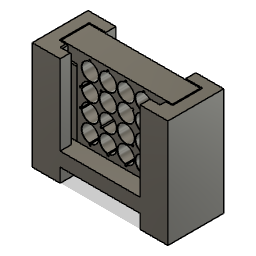
Prototype30 (Autodesk Fusion 360 design; units mm, degrees)
Autodesk Fusion 360 part; units mm, degrees
sketch "Esquisse1" plane through (0, 0, 0) normal (0, 0, 1) x (1, 0, 0) in component "Support_electroaimant"
  circle A0 centre (-16.1, 48.3478) radius 15.1
  line L0 (-14.9, 66.6) -> (-17.3, 66.6) construction
  line L1 (-17.3, 66.6) -> (-17.3, 63.4) construction
  line L2 (-17.3, 63.4) -> (-14.9, 63.4) construction
  line L3 (-14.9, 63.4) -> (-14.9, 66.6) construction
  line L4 (-14.9, 63.4) -> (-14.9, 66.6)
  line L5 (-17.3, 66.6) -> (-17.3, 63.4)
  line L6 (-14.9, 66.6) -> (-17.3, 66.6)
  line L7 (0, 71.8) -> (0, -71.8) construction
  line L8 (71.8, 71.8) -> (-71.8, 71.8)
  line L9 (-71.8, 71.8) -> (-71.8, -71.8)
  line L10 (-71.8, -71.8) -> (71.8, -71.8)
  line L11 (71.8, -71.8) -> (71.8, 71.8)
  line L12 (71.8, 71.8) -> (-71.8, -71.8) construction
  line L13 (-71.8, 71.8) -> (71.8, -71.8) construction
  line L14 (17.3, 63.4) -> (14.9, 63.4) construction
  line L15 (17.3, 66.6) -> (17.3, 63.4)
  line L16 (14.9, 66.6) -> (17.3, 66.6) construction
  line L17 (17.3, 66.6) -> (17.3, 63.4) construction
  line L18 (14.9, 63.4) -> (14.9, 66.6) construction
  line L19 (14.9, 63.4) -> (14.9, 66.6)
  line L20 (14.9, 66.6) -> (17.3, 66.6)
  circle A1 centre (16.1, 48.3478) radius 15.1
  line L21 (-32.2, 71.8) -> (-32.2, -71.8) construction
  line L22 (-47.1, 63.4) -> (-49.5, 63.4) construction
  line L23 (-49.5, 66.6) -> (-47.1, 66.6)
  line L24 (-47.1, 66.6) -> (-47.1, 63.4) construction
  circle A2 centre (-48.3, 48.3478) radius 15.1
  line L25 (-47.1, 66.6) -> (-47.1, 63.4)
  line L26 (-49.5, 63.4) -> (-49.5, 66.6)
  line L27 (-49.5, 63.4) -> (-49.5, 66.6) construction
  line L28 (-49.5, 66.6) -> (-47.1, 66.6) construction
  line L29 (32.2, 71.8) -> (32.2, -71.8) construction
  circle A3 centre (48.3, 48.3478) radius 15.1
  line L30 (49.5, 63.4) -> (49.5, 66.6) construction
  line L31 (47.1, 66.6) -> (47.1, 63.4)
  line L32 (49.5, 66.6) -> (47.1, 66.6) construction
  line L33 (47.1, 66.6) -> (47.1, 63.4) construction
  line L34 (47.1, 63.4) -> (49.5, 63.4) construction
  line L35 (49.5, 63.4) -> (49.5, 66.6)
  line L36 (49.5, 66.6) -> (47.1, 66.6)
  line L37 (-71.8, 0) -> (71.8, 0) construction
  circle A4 centre (-16.1, -48.3478) radius 15.1
  line L38 (-14.9, -66.6) -> (-17.3, -66.6)
  line L39 (-14.9, -63.4) -> (-14.9, -66.6)
  line L40 (47.1, -66.6) -> (47.1, -63.4)
  line L41 (47.1, -63.4) -> (49.5, -63.4) construction
  line L42 (-49.5, -66.6) -> (-47.1, -66.6)
  line L43 (17.3, -66.6) -> (17.3, -63.4) construction
  line L44 (17.3, -66.6) -> (17.3, -63.4)
  line L45 (14.9, -63.4) -> (14.9, -66.6) construction
  circle A5 centre (48.3, -48.3478) radius 15.1
  line L46 (49.5, -66.6) -> (47.1, -66.6)
  line L47 (49.5, -66.6) -> (47.1, -66.6) construction
  line L48 (17.3, -63.4) -> (14.9, -63.4) construction
  line L49 (-49.5, -63.4) -> (-49.5, -66.6) construction
  circle A6 centre (-48.3, -48.3478) radius 15.1
  circle A7 centre (16.1, -48.3478) radius 15.1
  line L50 (14.9, -63.4) -> (14.9, -66.6)
  line L51 (14.9, -66.6) -> (17.3, -66.6) construction
  line L52 (-49.5, -63.4) -> (-49.5, -66.6)
  line L53 (49.5, -63.4) -> (49.5, -66.6)
  line L54 (49.5, -63.4) -> (49.5, -66.6) construction
  line L55 (-17.3, -63.4) -> (-14.9, -63.4) construction
  line L56 (-14.9, -66.6) -> (-17.3, -66.6) construction
  line L57 (-49.5, -66.6) -> (-47.1, -66.6) construction
  line L58 (-47.1, -66.6) -> (-47.1, -63.4)
  line L59 (47.1, -66.6) -> (47.1, -63.4) construction
  line L60 (-14.9, -63.4) -> (-14.9, -66.6) construction
  line L61 (-17.3, -66.6) -> (-17.3, -63.4)
  line L62 (-47.1, -66.6) -> (-47.1, -63.4) construction
  line L63 (-17.3, -66.6) -> (-17.3, -63.4) construction
  line L64 (14.9, -66.6) -> (17.3, -66.6)
  line L65 (-47.1, -63.4) -> (-49.5, -63.4) construction
  line L66 (-71.8, 32.2478) -> (71.8, 32.2478) construction
  line L67 (-66.5522, 14.9478) -> (-63.3522, 14.9478) construction
  line L68 (-63.3522, 17.3478) -> (-66.5522, 17.3478) construction
  line L69 (-66.5522, 17.3478) -> (-66.5522, 14.9478) construction
  line L70 (-27.5921, 25.9428) -> (-29.8548, 28.2055)
  line L71 (-66.5522, 14.9478) -> (-63.3522, 14.9478)
  circle A8 centre (-16.1, 16.1478) radius 15.1
  line L72 (-63.3522, 17.3478) -> (-66.5522, 17.3478)
  line L73 (-25.895, 27.6398) -> (-27.5921, 25.9428) construction
  line L74 (-66.5522, 17.3478) -> (-66.5522, 14.9478)
  line L75 (-28.1578, 29.9026) -> (-25.895, 27.6398) construction
  line L76 (-29.8548, 28.2055) -> (-28.1578, 29.9026) construction
  line L77 (-63.3522, 14.9478) -> (-63.3522, 17.3478) construction
  line L78 (-27.5921, 25.9428) -> (-29.8548, 28.2055) construction
  circle A9 centre (-48.3, 16.1478) radius 15.1
  line L79 (-28.1578, 29.9026) -> (-25.895, 27.6398)
  line L80 (-29.8548, 28.2055) -> (-28.1578, 29.9026)
  line L81 (29.8548, 28.2055) -> (28.1578, 29.9026) construction
  line L82 (66.5522, 14.9478) -> (63.3522, 14.9478) construction
  line L83 (66.5522, 14.9478) -> (63.3522, 14.9478)
  circle A10 centre (48.3, 16.1478) radius 15.1
  line L84 (66.5522, 17.3478) -> (66.5522, 14.9478)
  line L85 (63.3522, 17.3478) -> (66.5522, 17.3478)
  line L86 (25.895, 27.6398) -> (27.5921, 25.9428) construction
  line L87 (27.5921, 25.9428) -> (29.8548, 28.2055) construction
  line L88 (28.1578, 29.9026) -> (25.895, 27.6398)
  line L89 (63.3522, 17.3478) -> (66.5522, 17.3478) construction
  circle A11 centre (16.1, 16.1478) radius 15.1
  line L90 (63.3522, 14.9478) -> (63.3522, 17.3478) construction
  line L91 (29.8548, 28.2055) -> (28.1578, 29.9026)
  line L92 (27.5921, 25.9428) -> (29.8548, 28.2055)
  line L93 (66.5522, 17.3478) -> (66.5522, 14.9478) construction
  line L94 (28.1578, 29.9026) -> (25.895, 27.6398) construction
  line L95 (66.5522, -17.3478) -> (66.5522, -14.9478) construction
  line L96 (-66.5522, -17.3478) -> (-66.5522, -14.9478) construction
  line L97 (-29.8548, -28.2055) -> (-28.1578, -29.9026)
  line L98 (-29.8548, -28.2055) -> (-28.1578, -29.9026) construction
  line L99 (-63.3522, -17.3478) -> (-66.5522, -17.3478)
  line L100 (-63.3522, -14.9478) -> (-63.3522, -17.3478) construction
  line L101 (-63.3522, -17.3478) -> (-66.5522, -17.3478) construction
  line L102 (-28.1578, -29.9026) -> (-25.895, -27.6398) construction
  line L103 (-66.5522, -17.3478) -> (-66.5522, -14.9478)
  line L104 (-25.895, -27.6398) -> (-27.5921, -25.9428) construction
  line L105 (29.8548, -28.2055) -> (28.1578, -29.9026)
  circle A12 centre (-48.3, -16.1478) radius 15.1
  line L106 (29.8548, -28.2055) -> (28.1578, -29.9026) construction
  line L107 (-66.5522, -14.9478) -> (-63.3522, -14.9478) construction
  line L108 (-27.5921, -25.9428) -> (-29.8548, -28.2055) construction
  circle A13 centre (-16.1, -16.1478) radius 15.1
  line L109 (-28.1578, -29.9026) -> (-25.895, -27.6398)
  line L110 (-27.5921, -25.9428) -> (-29.8548, -28.2055)
  line L111 (-66.5522, -14.9478) -> (-63.3522, -14.9478)
  line L112 (66.5522, -14.9478) -> (63.3522, -14.9478)
  line L113 (63.3522, -17.3478) -> (66.5522, -17.3478)
  line L114 (66.5522, -14.9478) -> (63.3522, -14.9478) construction
  line L115 (27.5921, -25.9428) -> (29.8548, -28.2055)
  circle A14 centre (16.1, -16.1478) radius 15.1
  line L116 (28.1578, -29.9026) -> (25.895, -27.6398)
  line L117 (63.3522, -17.3478) -> (66.5522, -17.3478) construction
  line L118 (25.895, -27.6398) -> (27.5921, -25.9428) construction
  circle A15 centre (48.3, -16.1478) radius 15.1
  line L119 (63.3522, -14.9478) -> (63.3522, -17.3478) construction
  line L120 (66.5522, -17.3478) -> (66.5522, -14.9478)
  line L121 (28.1578, -29.9026) -> (25.895, -27.6398) construction
  line L122 (27.5921, -25.9428) -> (29.8548, -28.2055) construction
  point P0 (-17.3, 63.4)
  point P1 (-14.9, 63.4)
  point P2 (-16.1, 66.6)
  point P3 (14.9, 63.4)
  point P4 (17.3, 63.4)
  point P5 (-1, 48.3478)
  point P6 (1, 48.3478)
  point P7 (-49.5, 63.4)
  point P8 (-47.1, 63.4)
  point P9 (-48.3, 66.6)
  point P10 (47.1, 63.4)
  point P11 (49.5, 63.4)
  point P12 (-63.4, -48.3478)
  point P13 (17.3, -63.4)
  point P14 (-48.3, -66.6)
  point P15 (49.5, -63.4)
  point P16 (14.9, -63.4)
  point P17 (-31.2, -48.3478)
  point P18 (1, -48.3478)
  point P19 (-16.1, -66.6)
  point P20 (-47.1, -63.4)
  point P21 (-1, -48.3478)
  point P22 (-14.9, -63.4)
  point P23 (-49.5, -63.4)
  point P24 (33.2, -48.3478)
  point P25 (31.2, -48.3478)
  point P26 (47.1, -63.4)
  point P27 (-17.3, -63.4)
  point P28 (-66.5522, 16.1478)
  point P29 (-63.3522, 14.9478)
  point P30 (-27.5921, 25.9428)
  point P31 (-29.0063, 29.054)
  point P32 (-25.895, 27.6398)
  point P33 (-63.3522, 17.3478)
  point P34 (27.5921, 25.9428)
  point P35 (66.5522, 16.1478)
  point P36 (63.3522, 14.9478)
  point P37 (63.3522, 17.3478)
  point P38 (71.8, 32.2478)
  point P39 (25.895, 27.6398)
  point P40 (29.0063, 29.054)
  point P41 (-25.895, -27.6398)
  point P42 (63.3522, -14.9478)
  point P43 (27.5921, -25.9428)
  point P44 (-66.5522, -16.1478)
  point P45 (25.895, -27.6398)
  point P46 (-63.3522, -14.9478)
  point P47 (-27.5921, -25.9428)
  point P48 (-63.3522, -17.3478)
  point P49 (63.3522, -17.3478)
  point P50 (66.5522, -16.1478)
  point P51 (-29.0063, -29.054)
  point P52 (29.0063, -29.054)
  dimension "d1" = 30.2
  dimension "d4" = 2.4
  dimension "d5" = 3.2
  dimension "d8" = 143.6
  dimension "d9" = 143.6
  dimension "d11" = 2
  dimension "d17" = 32.2
  dimension "d18" = 32.2
  dimension "d19" = 16.1
  constraint horizontal L0
  constraint vertical L1
  constraint horizontal L2
  constraint vertical L3
  constraint coincident P0 L1.end
  constraint coincident P1 L2.end
  constraint coincident A0 P0
  constraint coincident A0 P1
  constraint vertical L7
  constraint coincident origin L7
  constraint perpendicular L8 L9
  constraint parallel L8 L10
  constraint parallel L9 L11
  constraint coincident L12 origin
  constraint coincident L13 origin
  constraint midpoint L0 P2
  constraint symmetric A0 L7 A1
  constraint symmetric L0.start L7 L16.start
  constraint symmetric L0.end L7 L15.start
  constraint symmetric P0 L7 L14.start
  constraint symmetric P1 L7 P3
  constraint symmetric P0 L7 P4
  constraint coincident A0 P5
  constraint coincident A1 P6
  constraint vertical L21
  constraint symmetric A0 L21 A2
  constraint symmetric L0.start L21 L23.start
  constraint symmetric L0.end L21 L23.end
  constraint symmetric P0 L21 P8
  constraint symmetric P1 L21 P7
  constraint symmetric P1 L21 L22.end
  constraint symmetric P2 L21 P9
  constraint coincident L8 L21.start
  constraint coincident L10 L21.end
  constraint coincident L8 L29.start
  constraint coincident L10 L29.end
  constraint symmetric P3 L29 P11
  constraint symmetric P4 L29 P10
  constraint symmetric L15.start L29 L31.start
  constraint symmetric L16.start L29 L30.end
  constraint symmetric A1 L29 A3
  constraint symmetric A0 L37 A4
  constraint symmetric L0.start L37 L38.start
  constraint symmetric L0.end L37 L38.end
  constraint symmetric P0 L37 P27
  constraint symmetric P1 L37 P22
  constraint symmetric P2 L37 P19
  constraint symmetric P3 L37 L45.start
  constraint symmetric P4 L37 P13
  constraint symmetric P3 L37 P16
  constraint symmetric L15.start L37 L43.start
  constraint symmetric L16.start L37 L45.end
  constraint symmetric A1 L37 A7
  constraint symmetric P5 L37 P21
  constraint symmetric P6 L37 P18
  constraint symmetric P7 L37 P23
  constraint symmetric L23.end L37 L42.end
  constraint symmetric P8 L37 P20
  constraint symmetric P9 L37 P14
  constraint symmetric L23.start L37 L42.start
  constraint symmetric A2 L37 A6
  constraint symmetric P10 L37 P26
  constraint symmetric L30.end L37 L46.start
  constraint symmetric P11 L37 P15
  constraint symmetric L31.start L37 L40.start
  constraint symmetric A3 L37 A5
  constraint coincident L9 L66.start
  constraint coincident L11 P38
  constraint symmetric L7 L66.start P38
  constraint symmetric L7 L70.end L81.start
  constraint symmetric L7 L68.end L84.start
  constraint symmetric L7 P28 P35
  constraint symmetric L7 P29 P36
  constraint symmetric L7 P32 P39
  constraint symmetric L7 P33 P37
  constraint symmetric L7 L75.start L81.end
  constraint symmetric L7 P30 P34
  constraint symmetric L7 L67.start L82.start
  constraint symmetric L7 P31 P40
  constraint symmetric L7 A8 A11
  constraint symmetric L7 A9 A10
  constraint symmetric L37 L70.end L97.start
  constraint symmetric L37 L68.end L96.start
  constraint symmetric L37 P28 P44
  constraint symmetric L37 P29 P46
  constraint symmetric L37 P32 P41
  constraint symmetric L37 P33 P48
  constraint symmetric L37 L75.start L97.end
  constraint symmetric L37 P30 P47
  constraint symmetric L37 L67.start L96.end
  constraint symmetric L37 P31 P51
  constraint symmetric L37 A8 A13
  constraint symmetric L37 A9 A12
  constraint symmetric L37 P34 P43
  constraint symmetric L37 P36 P42
  constraint symmetric L37 P35 P50
  constraint symmetric L37 L82.start L95.end
  constraint symmetric L37 P37 P49
  constraint symmetric L37 L84.start L95.start
  constraint symmetric L37 L81.start L105.start
  constraint symmetric L37 P39 P45
  constraint symmetric L37 L81.end L105.end
  constraint symmetric L37 P40 P52
  constraint symmetric L37 A10 A15
  constraint symmetric L37 A11 A14
  measures "d1" diameter of A0
  measures "d4" distance of L0.start L0.end
  measures "d5" distance of L0.start P1
  measures "d8" distance of L8.end L9.end
  measures "d9" distance of L8.start L8.end
  measures "d11" distance of P5 P6
  measures "d17" distance of A0.centre A2.centre
  measures "d18" distance of A1.centre A3.centre
  measures "d19" distance of A2.centre L66
extrude "Extrusion2" add sketch "Esquisse1" against normal blind 25 contours A0 | L8 L9 L10 L11 | A1 | A2 | A3 | A4 | A5 | A6 | A7 | A8 | A9 | A10 | A11 | A13 | A12 | A14 | A15 makes body 1 in component "Support_electroaimant"
extrude "Extrusion1" add sketch "Esquisse1" along normal blind 25 bodies 1 in component "Support_electroaimant"
chamfer "Chanfrein1" distance 0.4 angle 45 64 edges at (-48.3, 66.6, 25) (-49.5, 65, 25) (-47.1, 65, 25) (-48.3, 33.2478, 25) (-16.1, 33.2478, 25) (-14.9, 65, 25) (-16.1, 66.6, 25) (-17.3, 65, 25) (16.1, 33.2478, 25) (14.9, 65, 25) (16.1, 66.6, 25) (17.3, 65, 25) (48.3, 33.2478, 25) (47.1, 65, 25) (48.3, 66.6, 25) (49.5, 65, 25) (33.2, 16.1478, 25) (64.9522, 17.3478, 25) (66.5522, 16.1478, 25) (64.9522, 14.9478, 25) (29.0063, 29.054, 25) (28.7234, 27.0741, 25) (27.0264, 28.7712, 25) (5.4227, 5.4704, 25) (-5.4227, 5.4704, 25) (-27.0264, 28.7712, 25) (-29.0063, 29.054, 25) (-28.7234, 27.0741, 25) (-33.2, 16.1478, 25) (-64.9522, 17.3478, 25) (-66.5522, 16.1478, 25) (-64.9522, 14.9478, 25) (-33.2, -16.1478, 25) (-64.9522, -14.9478, 25) (-66.5522, -16.1478, 25) (-64.9522, -17.3478, 25) (-5.4227, -5.4704, 25) (-28.7234, -27.0741, 25) (-29.0063, -29.054, 25) (-27.0264, -28.7712, 25) (5.4227, -5.4704, 25) (27.0264, -28.7712, 25) (29.0063, -29.054, 25) (28.7234, -27.0741, 25) (33.2, -16.1478, 25) (64.9522, -14.9478, 25) (66.5522, -16.1478, 25) (64.9522, -17.3478, 25) (48.3, -33.2478, 25) (47.1, -65, 25) (48.3, -66.6, 25) (49.5, -65, 25) (16.1, -33.2478, 25) (17.3, -65, 25) (16.1, -66.6, 25) (14.9, -65, 25) (-16.1, -33.2478, 25) (-14.9, -65, 25) (-16.1, -66.6, 25) (-17.3, -65, 25) (-48.3, -33.2478, 25) (-47.1, -65, 25) (-48.3, -66.6, 25) (-49.5, -65, 25) on bodies 1 in component "Support_electroaimant"
sketch "Esquisse2" plane through (-71.8, 0, 0) normal (-1, 0, 0) x (0, 0, 1) in component "Support_electroaimant"
  line L0 (25, 71.8) -> (-25, 71.8)
  line L1 (-25, 71.8) -> (-25, -71.8)
  line L2 (-25, -71.8) -> (25, -71.8)
  line L3 (-7.5, 71.8) -> (7.5, 71.8)
  line L4 (7.5, 71.8) -> (7.5, -71.8)
  line L5 (7.5, -71.8) -> (-7.5, -71.8)
  line L6 (-7.5, -71.8) -> (-7.5, 71.8)
  line L7 (-7.5, 71.8) -> (7.5, -71.8) construction
  line L8 (7.5, 71.8) -> (-7.5, -71.8) construction
  line L9 (-25, 71.8) -> (25, 71.8)
  line L10 (25, 71.8) -> (25, 46.8)
  line L11 (25, 46.8) -> (-25, 46.8)
  line L12 (-25, 46.8) -> (-25, 71.8)
  line L13 (25, -71.8) -> (25, 71.8)
  dimension "d24" = 50
  dimension "d25" = 25
  dimension "d26" = 15
  constraint horizontal L3
  constraint perpendicular L3 L4
  constraint parallel L3 L5
  constraint parallel L4 L6
  constraint coincident L7 origin
  constraint coincident L8 origin
  constraint horizontal L9
  constraint vertical L10
  constraint horizontal L11
  constraint vertical L12
  constraint coincident L0.end L1.start
  constraint collinear L3 L9
  measures "d24" distance of L0.end L0.start
  measures "d25" distance of L0.end L11.end
  measures "d26" distance of L3.start L3.end
extrude "Extrusion4" add sketch "Esquisse2" along normal blind 28 contours L0 L4 L9 L10 L11 L13 | L0 L3 L4 L6 L9 L11 | L0 L1 L6 L9 L11 L12 bodies 1 in component "Support_electroaimant"
chamfer "Chanfrein2" distance 2 angle 45 2 edges at (-85.8, 46.8, 25) (-85.8, 46.8, -25) on bodies 1 in component "Support_electroaimant"
extrude "Extrusion3" add sketch "Esquisse2" along normal blind 16 contours L2 L4 L5 L6 L11 bodies 1 in component "Support_electroaimant"
chamfer "Chanfrein3" distance 1 angle 45 4 edges at (-87.8, -12.5, -7.5) (-87.8, -12.5, 7.5) (-79.8, -71.8, 7.5) (-79.8, -71.8, -7.5) on bodies 1 in component "Support_electroaimant"
mirror "Symétrie miroir1" about plane through (0, 0, 0) normal (1, 0, 0) of "Extrusion4", "Extrusion3" in component "Support_electroaimant"
chamfer "Chanfrein4" distance 2 angle 45 2 edges at (85.8, 46.8, 25) (85.8, 46.8, -25) on bodies 1 in component "Support_electroaimant"
chamfer "Chanfrein5" distance 1 angle 45 4 edges at (87.8, -12.5, 7.5) (87.8, -12.5, -7.5) (79.8, -71.8, 7.5) (79.8, -71.8, -7.5) on bodies 1 in component "Support_electroaimant"
sketch "Esquisse2 (2)" plane through (-71.8, 0, 0) normal (-1, 0, 0) x (0, 0, 1) in component "Pieds"
  line L0 (-7.5, -70.8) -> (-7.5, 46.8)
  line L1 (-7.5, 46.8) -> (-23, 46.8)
  line L2 (-23, 46.8) -> (-25, 48.8)
  line L3 (-25, 48.8) -> (-25, -71.8)
  line L4 (-25, -71.8) -> (-6.5, -71.8)
  line L5 (-6.5, -71.8) -> (-7.5, -70.8)
  line L6 (-25, 71.8) -> (25, 71.8)
  line L7 (-25, 46.8) -> (-25, 71.8)
  line L8 (25, 46.8) -> (-25, 46.8)
  line L9 (25, 71.8) -> (25, 46.8)
  line L10 (-7.5, -71.8) -> (-7.5, 71.8)
  line L11 (7.5, 71.8) -> (7.5, -71.8)
  line L12 (7.5, -71.8) -> (-7.5, -71.8)
  line L13 (-25, -71.8) -> (-6.5, -71.8)
  line L14 (-25, -71.8) -> (-6.5, -71.8)
  line L15 (6.5, -71.8) -> (25, -71.8)
  line L16 (25, 48.8) -> (25, -71.8)
  line L17 (-25, -71.8) -> (-25, 48.8)
  line L18 (-25, 71.8) -> (-45, 71.8)
  line L19 (-45, 71.8) -> (-45, -71.8)
  line L20 (-45, -71.8) -> (-25, -71.8)
  line L21 (-25, -71.8) -> (-25, 71.8)
  line L22 (25, 71.8) -> (35.2, 71.8)
  line L23 (35.2, 71.8) -> (35.2, -71.8)
  line L24 (35.2, -71.8) -> (25, -71.8)
  line L25 (25, -71.8) -> (25, 71.8)
  line L26 (35.2, 71.8) -> (55.2, 71.8)
  line L27 (55.2, 71.8) -> (55.2, -71.8)
  line L28 (55.2, -71.8) -> (35.2, -71.8)
  line L29 (35.2, -71.8) -> (35.2, 71.8)
  line L30 (-45, -71.8) -> (55.2, -71.8)
  line L31 (55.2, -71.8) -> (55.2, -121.8)
  line L32 (55.2, -121.8) -> (-45, -121.8)
  line L33 (-45, -121.8) -> (-45, -71.8)
  dimension "d44" = 20
  dimension "d45" = 10.2
  dimension "d46" = 20
  dimension "d47" = 50
  constraint horizontal L18
  constraint vertical L19
  constraint horizontal L20
  constraint vertical L21
  constraint coincident L6.start L7.end
  constraint horizontal L22
  constraint vertical L23
  constraint horizontal L24
  constraint vertical L25
  constraint coincident L6.end L9.start
  constraint horizontal L26
  constraint vertical L27
  constraint horizontal L28
  constraint vertical L29
  constraint horizontal L30
  constraint vertical L31
  constraint horizontal L32
  constraint vertical L33
  measures "d44" distance of L6.start L18.end
  measures "d45" distance of L6.end L22.end
  measures "d46" distance of L22.end L26.end
  measures "d47" distance of L19.end L32.end
extrude "Extrusion6" add sketch "Esquisse2 (2)" along normal up to surface (16 mm away) separate body contours L0 L1 L3 L4 L8 L10 L13 L14 L17 L21 L30 | L4 L12 L13 L14 L15 L20 L24 L28 L30 L31 L32 L33 | L8 L11 L15 L16 L25 L30 | L3 L7 L17 L18 L19 L20 L21 L30 | L23 L26 L27 L28 L29 L30 makes body 2 in component "Pieds"
sketch "Esquisse6" plane through (-87.8, 0, 0) normal (-1, 0, 0) x (0, 0, 1) in component "Pieds"
  line L0 (35.2, -71.8) -> (25, -71.8)
  line L1 (25, -71.8) -> (25, 46.8)
  line L2 (25, 46.8) -> (7.5, 46.8)
  line L3 (7.5, 46.8) -> (7.5, -71.8)
  line L4 (7.5, -71.8) -> (-7.5, -71.8)
  line L5 (-7.5, -71.8) -> (-7.5, 46.8)
  line L6 (-7.5, 46.8) -> (-25, 46.8)
  line L7 (-25, 46.8) -> (-25, 71.8)
  line L8 (-25, 71.8) -> (-45, 71.8)
  line L9 (-45, 71.8) -> (-45, -121.8)
  line L10 (-45, -121.8) -> (55.2, -121.8)
  line L11 (55.2, -121.8) -> (55.2, 71.8)
  line L12 (55.2, 71.8) -> (35.2, 71.8)
  line L13 (35.2, 71.8) -> (35.2, -71.8)
  line L14 (-25, 71.8) -> (25, 71.8)
  line L15 (35.2, -71.8) -> (25, -71.8)
  line L16 (25, -71.8) -> (25, 71.8)
  line L17 (35.2, 71.8) -> (35.2, -71.8)
  line L18 (25, 71.8) -> (35.2, 71.8)
  line L19 (7.5, 71.8) -> (7.5, -71.8)
  line L20 (-7.5, -71.8) -> (-7.5, 71.8)
  line L21 (25, 46.8) -> (-25, 46.8)
  line L22 (-25, -71.8) -> (-25, 71.8)
extrude "Extrusion7" add sketch "Esquisse6" along normal up to surface (12 mm away) contours L0 L1 L2 L3 L4 L5 L6 L7 L8 L9 L10 L11 L12 L13 L15 L16 L17 L19 L20 L21 L22 | L0 L1 L13 L15 L16 L17 L18 | L3 L4 L5 L19 L20 L21 bodies 2 in component "Pieds"
sketch "Esquisse7" plane through (-99.8, 0, 0) normal (-1, 0, 0) x (0, 0, 1) in component "Pieds"
  line L0 (25, 71.8) -> (25, 46.8)
  line L1 (25, 46.8) -> (-25, 46.8)
  line L2 (-25, 46.8) -> (-25, 71.8)
  line L3 (-25, 71.8) -> (-45, 71.8)
  line L4 (-45, 71.8) -> (-45, -121.8)
  line L5 (-45, -121.8) -> (55.2, -121.8)
  line L6 (55.2, -121.8) -> (55.2, 71.8)
  line L7 (55.2, 71.8) -> (25, 71.8)
  line L8 (-45, 71.8) -> (55.2, 71.8)
  line L9 (55.2, 71.8) -> (55.2, -121.8)
  line L10 (55.2, -121.8) -> (-45, -121.8)
  line L11 (-45, -121.8) -> (-45, 71.8)
  constraint horizontal L8
  constraint vertical L9
  constraint horizontal L10
  constraint vertical L11
  constraint coincident L5.end L6.start
  constraint coincident L3.end L4.start
extrude "Extrusion8" add sketch "Esquisse7" along normal blind 22 bodies 2 in component "Pieds"
chamfer "Chanfrein5'" distance 2 angle 45 9 edges at (-79.8, 46.8, 25) (-79.8, 46.8, 7.5) (-87.8, 46.8, 0) (-79.8, 46.8, -7.5) (-79.8, 71.8, 35.2) (-87.8, 71.8, 30.1) (-93.8, 71.8, 25) (-93.8, 46.8, 25) (-85.8, 46.8, -25) on bodies 2 in component "Pieds"
chamfer "Chanfrein6" distance 2 angle 45 2 edges at (-85.8, 71.8, -25) (-99.8, 71.8, 1) on bodies 2 in component "Pieds"
mirror "Symétrie miroir2" about plane through (0, 0, 0) normal (1, 0, 0) of bodies 2 makes body 3 in component "Pieds"
sketch "Esquisse8" plane through (-71.8, 0, 0) normal (1, 0, 0) x (0, 0, -1) in component "Pieds"
  line L0 (27, 71.8) -> (25, 69.8)
  line L1 (25, 69.8) -> (25, 48.8)
  line L2 (25, 48.8) -> (23, 46.8)
  line L3 (23, 46.8) -> (9.5, 46.8)
  line L4 (9.5, 46.8) -> (7.5, 44.8)
  line L5 (7.5, 44.8) -> (7.5, -71.8)
  line L6 (7.5, -71.8) -> (-7.5, -71.8)
  line L7 (-7.5, -71.8) -> (-7.5, 44.8)
  line L8 (-7.5, 44.8) -> (-9.5, 46.8)
  line L9 (-9.5, 46.8) -> (-23, 46.8)
  line L10 (-23, 46.8) -> (-25, 44.8)
  line L11 (-25, 44.8) -> (-25, -71.8)
  line L12 (-25, -71.8) -> (-35.2, -71.8)
  line L13 (-35.2, -71.8) -> (-35.2, 69.8)
  line L14 (-35.2, 69.8) -> (-37.2, 71.8)
  line L15 (-37.2, 71.8) -> (-55.2, 71.8)
  line L16 (-55.2, 71.8) -> (-55.2, -121.8)
  line L17 (-55.2, -121.8) -> (45, -121.8)
  line L18 (45, -121.8) -> (45, 71.8)
  line L19 (45, 71.8) -> (27, 71.8)
  line L20 (-55.2, -71.8) -> (45, -71.8)
  line L21 (45, -71.8) -> (45, -121.8)
  line L22 (45, -121.8) -> (-55.2, -121.8)
  line L23 (-55.2, -121.8) -> (-55.2, -71.8)
  line L24 (-55.2, -96.8) -> (45, -96.8)
  line L25 (45, -96.8) -> (45, -121.8)
  line L26 (45, -121.8) -> (-55.2, -121.8)
  line L27 (-55.2, -121.8) -> (-55.2, -96.8)
  constraint horizontal L20
  constraint vertical L21
  constraint horizontal L22
  constraint vertical L23
  constraint coincident L17.end L18.start
  constraint coincident L16 L20.start
  constraint horizontal L24
  constraint vertical L25
  constraint horizontal L26
  constraint vertical L27
  constraint midpoint L23 L24.start
extrude "Extrusion9" add sketch "Esquisse8" along normal up to surface (143.6 mm away) contours L6 L12 L16 L18 L20 L21 L23 L24 bodies 2 3 in component "Pieds"
component "Support_electroaimant" placed x (1, 0, 0) y (0, 1, 0) z (0, 0, 1) at (0, 0, 0)
component "Pieds" placed x (1, 0, 0) y (0, 1, 0) z (0, 0, 1) at (0, 0, 0)
equation "d8 = 2 * d10 + 2 * d5 + 4 * d1 + ( 3 * 2 ) * 1 mm"
equation "d9 = d8"
equation "d10 = 5.2 mm"
equation "d17 = d1 + d11"
equation "d18 = d1 + d11"
equation "d19 = ( d1 + d11 ) / 2"
